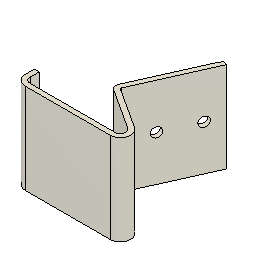
multimeterTiltBracketFluke101 (Autodesk Fusion 360 design; units mm, degrees)
Autodesk Fusion 360 part; units mm, degrees
note: some values were not read from the file. Set by a fixed rule: which sketch regions a step uses.
sketch "Sketch1" plane through (0, 0, 0) normal (0, 1, 0) x (1, 0, 0)
  arc A0 (31.1232, 52.6914) -> (20.5609, 48.637) centre (27.8693, 45.3831) ccw
  line L0 (31.1232, 52.6914) -> (40.2587, 48.6241)
  arc A1 (28.2837, -48.2895) -> (32.9132, -32.6608) centre (28.2837, -39.7895) ccw
  line L1 (28.2837, -48.2895) -> (-42.2163, -48.2895)
  arc A2 (-4.6567, -8.0029) -> (-2.8122, -14.2299) centre (-0.089, -10.0365) ccw
  line L2 (22.8004, 52.0184) -> (38.6317, 44.9699)
  line L3 (-46.7163, -32.2895) -> (-50.7163, -32.2895)
  line L4 (35.3386, -39.0053) -> (-23.3345, -39.0053) construction
  arc A3 (28.2837, -44.2895) -> (30.7346, -36.0155) centre (28.2837, -39.7895) ccw
  line L5 (40.2587, 48.6241) -> (38.6317, 44.9699)
  line L6 (30.7346, -36.0155) -> (-2.8122, -14.2299)
  line L7 (-50.7163, -39.7895) -> (-50.7163, -32.2895)
  line L8 (32.9132, -32.6608) -> (-0.6336, -10.8752)
  arc A4 (-46.7163, -39.7895) -> (-42.2163, -44.2895) centre (-42.2163, -39.7895) ccw
  arc A5 (-50.7163, -39.7895) -> (-42.2163, -48.2895) centre (-42.2163, -39.7895) ccw
  line L9 (-4.6567, -8.0029) -> (20.5609, 48.637)
  line L10 (28.2837, -44.2895) -> (-42.2163, -44.2895)
  line L11 (-46.7163, -39.7895) -> (-46.7163, -32.2895)
  arc A6 (22.8004, 52.0184) -> (27.1963, 53.7059) centre (27.8693, 45.3831) ccw
  arc A7 (-1.0025, -9.6298) -> (-0.6336, -10.8752) centre (-0.089, -10.0365) ccw
  line L12 (-1.0025, -9.6298) -> (27.1963, 53.7059)
  point P0 (35.3386, -39.0053)
  point P1 (-46.7163, -44.2895)
  point P2 (23.8148, 55.9453)
  dimension "d1" = 33
  dimension "d2" = 66
  dimension "d3" = 4.5
  dimension "d4" = 5
  dimension "d5" = 12
  dimension "d6" = 18
  dimension "d10" = 75
  dimension "d11" = 70
  dimension "d12" = 40
  dimension "d13" = 8
  dimension "d14" = 4.5
  constraint coincident P0 L4.start
  constraint coincident P0 L6
  constraint tangent A3 L10
  constraint tangent A3 L6
  constraint tangent A2 L6
  constraint tangent A2 L9
  constraint perpendicular L10 L11
  constraint perpendicular L0 L9
  constraint coincident P2 L9
  constraint coincident P2 L0
  constraint tangent A0 L9
  constraint tangent A0 L0
  constraint coincident P1 L10
  constraint coincident P1 L11
  constraint tangent A4 L10
  constraint tangent A4 L11
  constraint concentric A4 A5
  constraint concentric A1 A3
  constraint concentric A2 A7
  constraint concentric A0 A6
  constraint tangent L7 A5
  constraint tangent A1 L8
  constraint tangent L1 A5
  constraint tangent A1 L1
  constraint tangent L8 A7
  constraint tangent A7 L12
  measures "d1" angle of L4 L6
  measures "d2" angle of L4 L9
  measures "d3" radius of A3
  measures "d4" radius of A2
  measures "d5" distance of P1 L3.start
  measures "d6" distance of P2 L0.end
  measures "d10" distance of P1 A3.start
  measures "d11" distance of A2.start P2
  measures "d12" distance of A3.end A2.end
  measures "d13" radius of A0
  measures "d14" radius of A4
extrude "Extrude1" add sketch "Sketch1" along normal blind 75 contours A0 L2 L9 A6 L12 | A1 L1 A2 L3 A3 L6 L7 L8 A4 A5 L9 L10 L11 A6 A7 L12
sketch "Sketch2" plane through (-0.9127, 0, -0.4064) normal (-0.913545, 0, -0.406737) x (-0.406737, 0, 0.913545)
  line L0 (-52.795, 0) -> (9.205, 0)
  line L1 (9.205, 0) -> (9.205, 75)
  line L2 (9.205, 75) -> (-52.795, 75)
  line L3 (-52.795, 75) -> (-52.795, 0)
  circle A0 centre (-42.795, 37.5) radius 4
  circle A1 centre (-12.795, 37.5) radius 4
  line L4 (-31.6238, 0) -> (-31.6238, 75)
  line L5 (9.205, 37.5) -> (-64.6996, 37.5)
  dimension "d17" = 8
  dimension "d18" = 8
  dimension "d23" = 10
  dimension "d24" = 30
  constraint coincident L0 L4.start
  constraint coincident L2 L4.end
  constraint perpendicular L2 L4
  constraint perpendicular L4 L5
  constraint coincident L1 L5.start
  constraint coincident A0.centre L5
  constraint coincident A1.centre L5
  measures "d17" diameter of A0
  measures "d18" diameter of A1
  measures "d23" distance of L3 A0.centre
  measures "d24" distance of A0.centre A1.centre
extrude "Extrude2" cut sketch "Sketch2" along normal blind 18 and the other way blind 25 contours A0 L5 | A0 L5 | A1 L5 | A1 L5
